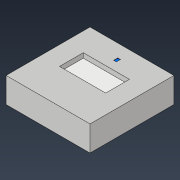
# Autodesk Inventor part: iC-PX Series Encoder
Saved by Autodesk Inventor 2022.1 (Build 261234020, 234B)
## iProperties
Part Number: iC-PX Series Encoder
Material: Generisch
Document SubType Name: Modeling
Designer: rYan
Density: 1 g/cm^3
Appearance: Vorgabe
Mass: 0.00786128 g
Surface Area: 0.2966 cm^2
Volume: 0.00786128 cm^3
Author: rYan
Autodesk Inventor part; units mm, degrees
ref_plane "YZ Plane" through (0, 0, 0) normal (1, 0, 0) x (0, 1, 0)
ref_plane "XZ Plane" through (0, 0, 0) normal (0, 1, 0) x (-1, 0, 0)
ref_plane "XY Plane" through (0, 0, 0) normal (0, 0, 1) x (1, 0, 0)
sketch "Skizze1" plane through (0, 0, 0) normal (0, 0, 1) x (1, 0, 0)
  line L0 (-1.5, -1.5) -> (1.5, -1.5)
  line L1 (1.5, -1.5) -> (1.5, 1.5)
  line L2 (1.5, 1.5) -> (-1.5, 1.5)
  line L3 (-1.5, 1.5) -> (-1.5, -1.5)
  line L4 (-1.5, -1.5) -> (1.5, 1.5) construction
  line L5 (1.5, -1.5) -> (-1.5, 1.5) construction
  point P0 (0, 0)
  dimension "d0" = 3
  dimension "d1" = 3
  constraints: 12 end point, 2 midpoint, 2 parallel, 1 horizontal, 1 perpendicular
  measures "d0" distance of L2.end L1.end
  measures "d1" distance of L1.end L0.end
extrude "Extrusion1" add sketch "Skizze1" along normal blind 0.9
sketch "Skizze2" plane through (0, 0, 0.9) normal (0, 0, 1) x (1, 0, 0)
  line L0 (-0.825, 0.585) -> (0.825, 0.585)
  line L1 (0.825, 0.585) -> (0.825, -0.265)
  line L2 (0.825, -0.265) -> (-0.825, -0.265)
  line L3 (-0.825, -0.265) -> (-0.825, 0.585)
  line L4 (-0.825, 0.585) -> (0.825, -0.265) construction
  line L5 (0.825, 0.585) -> (-0.825, -0.265) construction
  line L6 (0, 2.1) -> (0, -2.1) projected
  point P0 (0, 0)
  point P1 (0, 0.16)
  point P2 (0, 0.16)
  dimension "d4" = 1.65
  dimension "d5" = 0.85
  dimension "d6" = 0.16
  constraints: 12 end point, 3 midpoint, 2 parallel, 1 horizontal, 1 perpendicular, 1 point on line
  measures "d4" distance of L0.start L0.end
  measures "d5" distance of L0.end L1.end
  measures "d6" distance of point (0, 0.16) point (0, 0)
extrude "Extrusion2" cut sketch "Skizze2" against normal blind 0.17
sketch "Skizze3" plane through (0, 0, 0.9) normal (0, 0, 1) x (1, 0, 0)
  line L0 (0, 2.1) -> (0, -2.1) projected
  line L1 (-0.05, 1.042) -> (0.05, 1.042)
  line L2 (0.05, 1.042) -> (0.05, 0.892)
  line L3 (0.05, 0.892) -> (-0.05, 0.892)
  line L4 (-0.05, 0.892) -> (-0.05, 1.042)
  line L5 (-0.05, 1.042) -> (0.05, 0.892) construction
  line L6 (0.05, 1.042) -> (-0.05, 0.892) construction
  point P0 (0, 0)
  point P1 (0, 0.967)
  dimension "d9" = 0.967
  dimension "d10" = 0.1
  dimension "d11" = 0.15
  constraints: 12 end point, 2 midpoint, 2 parallel, 1 horizontal, 1 perpendicular, 1 point on line
  measures "d9" distance of point (0, 0.967) point (0, 0)
  measures "d10" distance of L1.start L1.end
  measures "d11" distance of L1.end L2.end
extrude "Extrusion3" cut sketch "Skizze3" against normal blind 0.02
